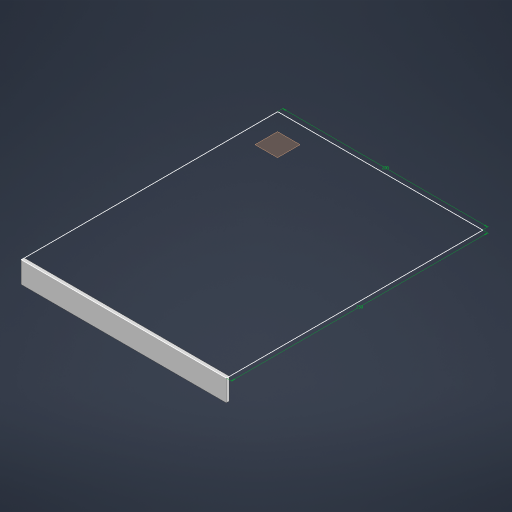
# Autodesk Inventor part: side_left
Saved by Autodesk Inventor 2023 (Build 270158000, 158)
## iProperties
Created: 2022-12-04
Part Number: side_left
Material: Glass
Document SubType Name: Modeling
Designer: jeff7
Density: 2.18 g/cm^3
Appearance: Default
Author: jeff7
Autodesk Inventor part; units mm, degrees
ref_plane "YZ Plane" through (0, 0, 0) normal (1, 0, 0) x (0, 1, 0)
ref_plane "XZ Plane" through (0, 0, 0) normal (0, 1, 0) x (-1, 0, 0)
ref_plane "XY Plane" through (0, 0, 0) normal (0, 0, 1) x (1, 0, 0)
sketch "block" plane through (0, 0, 0) normal (0, 1, 0) x (-1, 0, 0)
  line L0 (0, 0) -> (-200, 0)
  line L1 (-200, 0) -> (-200, -250)
  line L2 (-200, -250) -> (0, -250)
  line L3 (0, -250) -> (0, 0)
  dimension "d31" = 200
  dimension "d32" = 250
  constraints: 8 end point, 2 parallel, 1 horizontal, 1 perpendicular
  measures "d31" distance of L2.end L1.end
  measures "d32" distance of L1.end L0.end
extrude "ext_block" add sketch "block" against normal blind 24
shell "Shell2" thickness 3 removed faces 0
sketch "lines_base" plane through (0, 0, 0) normal (0, 1, 0) x (-1, 0, 0)
  line L0 (0, 0) -> (-200, 0)
  line L1 (-200, 0) -> (-200, -250)
  line L2 (-200, -250) -> (0, -250)
  line L3 (0, -250) -> (0, 0)
  circle A0 centre (-65, -60) radius 6
  circle A1 centre (-125, -80) radius 6
  circle A2 centre (-65, -60) radius 12.5
  circle A3 centre (-65, -60) radius 8.5
  circle A4 centre (-125, -80) radius 8.5
  circle A5 centre (-125, -80) radius 12.5
  circle A6 centre (-175, -125) radius 3
  line L4 (-175, -125) -> (-175, -209)
  line L5 (-175, -125) -> (-91, -125) construction
  circle A7 centre (-175, -139) radius 3
  circle A8 centre (-175, -153) radius 3
  circle A9 centre (-175, -167) radius 3
  circle A10 centre (-175, -181) radius 3
  circle A11 centre (-175, -195) radius 3
  circle A12 centre (-175, -209) radius 3
  circle A13 centre (-95, -185) radius 2.5
  circle A14 centre (-95, -185) radius 5
  point P0 (-200, -125)
  dimension "d0" = 200
  dimension "d1" = 250
  dimension "d2" = 12
  dimension "d3" = 12
  dimension "d4" = 25
  dimension "d5" = 17
  dimension "d6" = 17
  dimension "d7" = 25
  dimension "d8" = 75
  dimension "d9" = 80
  dimension "d10" = 65
  dimension "d11" = 60
  dimension "d12" = 6
  dimension "d13" = 84
  dimension "d14" = 90
  dimension "d15" = 25
  dimension "d16" = 125
  dimension "d19" = 14
  dimension "d24" = 5
  dimension "d25" = 10
  dimension "d26" = 65
  dimension "d27" = 95
  constraints: 15 centre point, 12 end point, 5 coincident, 2 horizontal, 2 parallel, 2 perpendicular, 2 vertical, 1 midpoint, 12 other
  measures "d0" distance of L2.end L1.end
  measures "d1" distance of L1.end L0.end
  measures "d2" diameter of A0
  measures "d3" diameter of A1
  measures "d4" diameter of A2
  measures "d5" diameter of A3
  measures "d6" diameter of A4
  measures "d7" diameter of A5
  measures "d8" distance from line of L1 A1.centre
  measures "d9" distance from line of L0 A1.centre
  measures "d10" distance from line of L3 A0.centre
  measures "d11" distance from line of L0 A0.centre
  measures "d12" diameter of A6
  measures "d13" distance of L4.start L4.end
  measures "d14" angle of L4 L5
  measures "d15" distance of point (-200, -125) L4.start
  measures "d16" distance from line of L0 L4.start
  measures "d19" distance of L4.start A7.centre
  measures "d24" diameter of A13
  measures "d25" diameter of A14
  measures "d26" distance from line of L2 A13.centre
  measures "d27" distance from line of L3 A13.centre
extrude "holes" cut sketch "lines_base" against normal up to surface (3 mm away) contours A0 | A1 | A6 | A7 L4 | L4 A7 | A8 L4 | L4 A8 | A9 L4 | L4 A9 | A10 L4 | L4 A10 | A11 L4 | L4 A11 | A12 | A13
sketch "Sketch4" plane through (200, 0, -250) normal (0, 0, -1) x (-1, 0, 0)
  line L0 (188, -4) -> (169, -4)
  line L1 (169, -4) -> (169, -17)
  line L2 (169, -17) -> (188, -17)
  line L3 (188, -17) -> (188, -4)
  line L4 (0, 0) -> (200, 0) projected
  line L5 (200, 0) -> (200, -24) projected
  dimension "d40" = 19
  dimension "d41" = 13
  dimension "d42" = 4
  dimension "d43" = 12
  constraints: 8 end point, 2 parallel, 1 horizontal, 1 perpendicular
  measures "d40" distance of L2.end L1.end
  measures "d41" distance of L1.end L0.end
  measures "d42" distance between parallel lines of L4 L0
  measures "d43" distance between parallel lines of L5 L3
extrude "pwr_button_hole" cut sketch "Sketch4" against normal up to surface (3 mm away)
ref_plane "Work Plane1" through (7, -21, -243) normal (0, 1, 0) x (1, 0, 0)
sketch "Sketch5" plane through (7, -21, -243) normal (0, 1, 0) x (1, 0, 0)
  line L0 (-20.9366, 21.7948) -> (229.9216, 21.7948)
  line L1 (229.9216, 21.7948) -> (229.9216, -260.9184)
  line L2 (229.9216, -260.9184) -> (-20.9366, -260.9184)
  line L3 (-20.9366, -260.9184) -> (-20.9366, 21.7948)
  point P0 (-7, -243)
  constraints: 8 end point, 2 parallel, 1 horizontal, 1 perpendicular
extrude "back_cover_cut" cut sketch "Sketch5" against normal through all
sketch "Sketch8" plane through (197, -3, -3) normal (0, 0, -1) x (-1, 0, 0)
  line L0 (-20.5673, 18.4526) -> (237.6144, 18.4526)
  line L1 (237.6144, 18.4526) -> (237.6144, -33.7854)
  line L2 (237.6144, -33.7854) -> (-20.5673, -33.7854)
  line L3 (-20.5673, -33.7854) -> (-20.5673, 18.4526)
  point P0 (197, 3)
  constraints: 8 end point, 2 parallel, 1 horizontal, 1 perpendicular
extrude "Extrusion8" cut sketch "Sketch8" along normal through all
body "Solid3"
